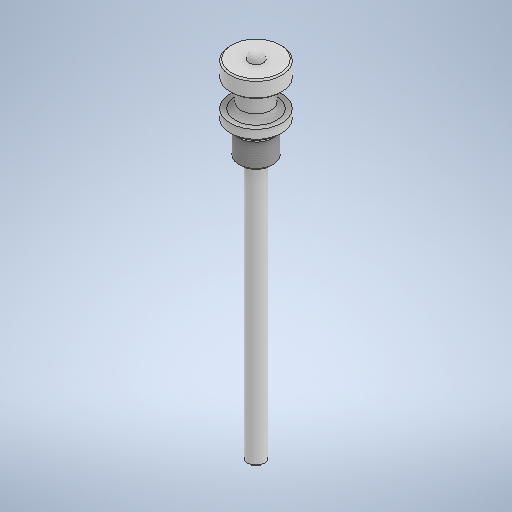
# Autodesk Inventor part: 05_Que_tham_dau
Saved by Autodesk Inventor 2025.2 (Build 292293000, 293)
## iProperties
Created: 2024-11-26
Part Number: 05_Que_tham_dau
Material: Generic
Document SubType Name: Modeling
Designer: hongquan
Density: 1 g/cm^3
Appearance: Default
Author: hongquan
Autodesk Inventor part; units mm, degrees
ref_plane "YZ Plane" through (0, 0, 0) normal (1, 0, 0) x (0, 1, 0)
ref_plane "XZ Plane" through (0, 0, 0) normal (0, 1, 0) x (-1, 0, 0)
ref_plane "XY Plane" through (0, 0, 0) normal (0, 0, 1) x (1, 0, 0)
sketch "Sketch1" plane through (0, 0, 0) normal (1, 0, 0) x (0, 1, 0)
  line L0 (0, 0) -> (124.5, 0)
  line L1 (0, 0) -> (92, 0)
  line L2 (92, 0) -> (92, 3)
  line L3 (92, 3) -> (0, 3)
  line L4 (0, 3) -> (0, 0)
  line L5 (92, 0) -> (101, 0)
  line L6 (101, 0) -> (101, 6)
  line L7 (101, 6) -> (92, 6)
  line L8 (92, 6) -> (92, 0)
  line L9 (101, 0) -> (103, 0)
  line L10 (103, 0) -> (103, 5.25)
  line L11 (103, 5.25) -> (101, 5.25)
  line L12 (101, 5.25) -> (101, 0)
  line L13 (103, 0) -> (107, 0)
  line L14 (107, 0) -> (107, 9)
  line L15 (107, 9) -> (103, 9)
  line L16 (103, 9) -> (103, 0)
  line L17 (107, 0) -> (116, 0)
  line L18 (116, 0) -> (116, 5.25)
  line L19 (116, 5.25) -> (107, 5.25)
  line L20 (107, 5.25) -> (107, 0)
  line L21 (116, 0) -> (122, 0)
  line L22 (122, 0) -> (122, 9)
  line L23 (122, 9) -> (116, 9)
  line L24 (116, 9) -> (116, 0)
  arc A0 (124.5, 0) -> (122, 2.5) centre (122, 0) ccw
  dimension "d0" = 6
  dimension "d2" = 12
  dimension "d3" = 9
  dimension "d5" = 2
  dimension "d6" = 92
  dimension "d7" = 10.5
  dimension "d8" = 18
  dimension "d9" = 4
  dimension "d10" = 9
  dimension "d11" = 6
  dimension "d12" = 5
  constraints: 51 end point, 12 parallel, 8 horizontal, 6 perpendicular, 2 collinear, 2 point on circle, 1 centre point, 1 coincident, 1 point on line
  measures "d0" diameter of L3 L0
  measures "d2" diameter of L7 L0
  measures "d3" distance of L6.end L7.end
  measures "d5" distance of L10.end L11.end
  measures "d6" distance of L2.end L3.end
  measures "d7" diameter of L11 L0
  measures "d8" diameter of L15 L0
  measures "d9" distance of L14.end L15.end
  measures "d10" distance of L18.end L19.end
  measures "d11" distance of L22.end L23.end
  measures "d12" diameter of A0
revolve "Revolution1" add sketch "Sketch1" angle 360 about axis through (0, 0, 0) along (0, 1, 0)
chamfer "Chamfer1" distance 1 angle 45 1 edges at (0, 0, -3)
chamfer "Chamfer2" distance 1 angle 45 1 edges at (0, 92, -6)
chamfer "Chamfer3" distance 1 angle 45 1 edges at (0, 103, -9)
chamfer "Chamfer4" distance 0.5 angle 45 2 edges at (0, 122, -9) (0, 116, -9)
fillet "Fillet1" radius 2 2 edges at (0, 107, -5.25) (0, 116, -5.25)
thread "Thread1" size "M12x0.5" class "6g" standard "ISO Metric profile" full length
body "Solid1"
